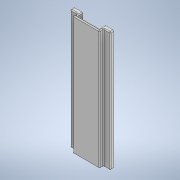
# Autodesk Inventor part: CableCover
Saved by Autodesk Inventor 2021.3 (Build 253353000, 353)
## iProperties
Created: 2021-05-14
Part Number: CableCover
Material: 一般
Document SubType Name: Modeling
Designer: gisen
Density: 1 g/cm^3
Appearance: 既定
Author: gisen
Autodesk Inventor part; units mm, degrees
ref_plane "YZ Plane" through (0, 0, 0) normal (1, 0, 0) x (0, 1, 0)
sketch "スケッチ1" plane through (0, 0, 0) normal (0, 0, 1) x (1, 0, 0)
  line L0 (0, 0) -> (60, 0)
  line L1 (60, 0) -> (60, 270)
  line L2 (60, 270) -> (0, 270)
  line L3 (0, 270) -> (0, 0)
  dimension "d0" = 270
  dimension "d1" = 60
  constraints: 8 end point, 2 parallel, 1 horizontal, 1 perpendicular
  measures "d0" distance of L2.end L0.start
  measures "d1" distance of L0.start L0.end
extrude "押し出し1" add sketch "スケッチ1" along normal blind 17
ref_plane "作業平面1" through (30, 0, 0) normal (1, 0, 0) x (0, 0, -1)
ref_plane "作業平面2" through (0, 135, 0) normal (0, -1, 0) x (1, 0, 0)
sketch "スケッチ2" plane through (0, 0, 0) normal (0, -1, 0) x (1, 0, 0)
  line L0 (30, 24) -> (30, -4) projected
  line L1 (60, 0) -> (0, 0) projected
  line L2 (30, 0) -> (5, 0)
  line L3 (5, 0) -> (5, 12)
  line L4 (5, 12) -> (30, 12)
  line L5 (30, 12) -> (30, 0)
  line L6 (0, 17) -> (60, 17) projected
  line L7 (0, 0) -> (0, 17) projected
  line L8 (55, 0) -> (55, 12)
  line L9 (55, 12) -> (30, 12)
  point P0 (5, 0)
  dimension "d4" = 5
  dimension "d5" = 5
  constraints: 12 end point, 2 parallel, 2 symmetric about line, 1 horizontal, 1 midpoint, 1 perpendicular
  measures "d4" distance between parallel lines of L6 L4
  measures "d5" distance between parallel lines of L7 L3
extrude "押し出し2" cut sketch "スケッチ2" against normal through all contours L9 L8 L1 L0 | L0 L1 L3 L4
sketch "スケッチ3" plane through (0, 0, 17) normal (0, -1, 0) x (1, 0, 0)
  line L0 (5, -17) -> (0, -17) projected
  line L1 (0, -17) -> (-15, -17)
  line L2 (-15, -17) -> (-15, -9)
  line L3 (-15, -9) -> (0, -9)
  line L4 (0, -9) -> (0, -17)
  line L5 (30, 3.4) -> (30, -20.4) projected
  line L6 (60, -17) -> (75, -17)
  line L7 (75, -17) -> (75, -9)
  line L8 (75, -9) -> (60, -9)
  line L9 (60, -9) -> (60, -17)
  dimension "d8" = 8
  dimension "d9" = 15
  constraints: 16 end point, 4 symmetric about line, 2 parallel, 1 horizontal, 1 perpendicular
  measures "d8" distance of L3.end L0.end
  measures "d9" distance of L0.end L1.end
extrude "押し出し3" add sketch "スケッチ3" against normal up to surface (270 mm away)
sketch "スケッチ4" plane through (0, 0, 0) normal (0, 0, 1) x (1, 0, 0)
  line L0 (-15, 0) -> (5, 0) projected
  line L1 (-15, 0) -> (-15, 270) projected
  line L2 (30, 324) -> (30, -54) projected
  line L3 (93, 135) -> (-33, 135) projected
  point P0 (0, 0)
  point P1 (-7.5, 60)
  point P2 (-7.5, 210)
  point P3 (67.5, 60)
  point P4 (67.5, 210)
  dimension "d12" = 60
  dimension "d13" = 7.5
  constraints: 3 symmetric about line
  measures "d12" distance from line of L0 point (-7.5, 60)
  measures "d13" distance from line of L1 point (-7.5, 60)
hole "穴1" at (-7.5, 60, 0) at (-7.5, 210, 0) at (67.5, 60, 0) at (67.5, 210, 0) direction (0, 0, 1) diameter 3.3 depth 5 tip angle 118
fillet "フィレット1" radius 2 26 edges at (30, 0, 17) (30, 0, 12) (5, 0, 6) (55, 0, 6) (60, 0, 12.5) (60, 135, 17) (67.5, 0, 8) (75, 0, 4) (75, 135, 8) (0, 0, 12.5) (-7.5, 0, 8) (-15, 135, 8) (-15, 0, 4) (0, 135, 17) (0, 135, 8) (60, 135, 8) (30, 270, 17) (0, 270, 12.5) (60, 270, 12.5) (67.5, 270, 8) (-7.5, 270, 8) (75, 270, 4) (-15, 270, 4) (30, 270, 12) (55, 270, 6) (5, 270, 6)
